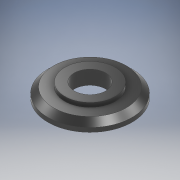
# Autodesk Inventor part: x carraige sliding spacer short
Saved by Autodesk Inventor 2020.2 (Build 242310000, 310)
## iProperties
Created: 2019-11-18
Part Number: x carraige sliding spacer short
Material: ABS Plastic
Document SubType Name: Modeling
Designer: Richard Hall
Density: 1.06 g/cm^3
Appearance: Satin - Black
Author: Richard Hall
Autodesk Inventor part; units mm, degrees
ref_plane "YZ Plane" through (0, 0, 0) normal (1, 0, 0) x (0, 1, 0)
ref_plane "XZ Plane" through (0, 0, 0) normal (0, 1, 0) x (-1, 0, 0)
ref_plane "XY Plane" through (0, 0, 0) normal (0, 0, 1) x (1, 0, 0)
sketch "Sketch1" plane through (0, 0, 0) normal (0, 1, 0) x (-1, 0, 0)
  circle A0 centre (0, 0) radius 2.8
  circle A1 centre (0, 0) radius 7.5
  dimension "d0" = 5.6
  dimension "d1" = 15
  constraints: 2 centre point, 2 coincident
  measures "d0" diameter of A0
  measures "d1" diameter of A1
extrude "Extrusion1" add sketch "Sketch1" along normal blind 1.75
sketch "Sketch2" plane through (0, 1.75, 0) normal (0, 1, 0) x (1, 0, 0)
  circle A0 centre (0, 0) radius 4.5
  circle A1 centre (0, 0) radius 2.8 projected
  dimension "d4" = 9
  constraints: 1 centre point, 1 coincident
  measures "d4" diameter of A0
extrude "Extrusion2" add sketch "Sketch2" along normal blind 0.75
chamfer "Chamfer1" distance 1 angle 45 1 edges at (7.5, 1.75, 0)
body "Solid1"
